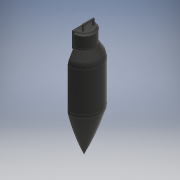
# Autodesk Inventor part: noze-cone
Saved by Autodesk Inventor 2017 (Build 210142000, 142)
## iProperties
Created: 2020-06-18
Part Number: noze-cone
Material: Polycarbonate, Clear
Document SubType Name: Modeling
Designer: HAYNIE R&D
Density: 1.2 g/cm^3
Appearance: Smooth - Black
Mass: 19.1961 g
Surface Area: 332.143 cm^2
Volume: 18.1095 cm^3
Author: HAYNIE R&D
Autodesk Inventor part; units mm, degrees
ref_plane "YZ Plane" through (0, 0, 0) normal (1, 0, 0) x (0, 1, 0)
ref_plane "XZ Plane" through (0, 0, 0) normal (0, 1, 0) x (-1, 0, 0)
ref_plane "XY Plane" through (0, 0, 0) normal (0, 0, 1) x (1, 0, 0)
sketch "Sketch1" plane through (0, 0, 0) normal (1, 0, 0) x (0, 1, 0)
  line L0 (0, 0) -> (0, -200)
  line L1 (17.75, -33.271) -> (27.75, -50.5915)
  line L2 (27.75, -50.5915) -> (27.75, -125.5915)
  line L3 (16.75, -33.271) -> (26.75, -50.5915)
  line L4 (16.75, -33.271) -> (36.75, -33.271) construction
  line L5 (26.75, -50.5915) -> (26.75, -125.5915)
  line L6 (17.75, -33.271) -> (17.75, -13.271)
  line L7 (16.75, -13.271) -> (32.074, -13.271) construction
  line L8 (17.75, -13.271) -> (33.074, -13.271) construction
  line L9 (17.75, -13.271) -> (33.074, -13.271) construction
  line L10 (16.75, -13.271) -> (31.4966, -13.271) construction
  line L11 (16.75, -33.271) -> (16.75, -14.271)
  line L12 (16.75, -14.271) -> (0, -14.271)
  line L13 (17.75, -13.271) -> (0, -13.271)
  arc A0 (0, -200) -> (27.75, -125.5915) centre (-356.6732, -24.6031) ccw
  line L14 (0, -200) -> (0, -199)
  arc A1 (0, -199) -> (26.75, -125.5915) centre (-482.9464, 18.5633) ccw
  line L15 (0, -200) -> (0, -199)
  point P0 (0, -1)
  dimension "d0" = 200
  dimension "d7" = 75
  dimension "d31" = 19
  constraints: 32 end point, 5 horizontal, 5 point on line, 5 vertical, 4 point on circle, 2 centre point, 1 collinear, 1 equal length, 1 perpendicular
  measures "d0" distance of L0.start L0.end
  measures "d7" distance of L1.end L2.end
  measures "d31" distance of L3.start L11.end
revolve "Revolution2" add sketch "Sketch1" angle 360 about axis through (0, 0, 0) along (0, 0, -1) contours L13 L6 L1 L2 A0 L0 A1 L5 L3 L11 L12
fillet "Fillet5" radius 5 1 edges at (0, -17.75, -33.271)
sketch "Sketch4" plane through (0, 0, -13.271) normal (0, 0, 1) x (1, 0, 0)
  circle A0 centre (0, 0) radius 15
  dimension "d36" = 30
  constraints: 1 centre point, 1 coincident
  measures "d36" diameter of A0
extrude "Extrusion2" add sketch "Sketch4" along normal blind 3.27
split "Split3" plane through (0, 0, 0) removes the side toward (-1, 0, 0)
fillet "Fillet8" radius 20 1 edges at (27.75, 0, -50.5915)
fillet "Fillet9" radius 25 1 edges at (27.75, 0, -125.5915)
fillet "Fillet10" radius 10 1 edges at (15, 0, -13.271)
sketch "Sketch8" plane through (0, 0, -10.001) normal (0, 0, 1) x (1, 0, 0)
  line L0 (8, -10) -> (6, -10)
  line L1 (6, -10) -> (6, -8)
  line L2 (6, -8) -> (8, -8)
  line L3 (8, -8) -> (8, -10)
  line L4 (8, 8) -> (6, 8)
  line L5 (6, 8) -> (6, 10)
  line L6 (6, 10) -> (8, 10)
  line L7 (8, 10) -> (8, 8)
  point P0 (0, 0)
  dimension "d49" = 16
  constraints: 16 end point, 4 parallel, 2 horizontal, 2 perpendicular
  measures "d49" distance of L4.end L1.end
extrude "Extrusion5" add sketch "Sketch8" along normal blind 10
sketch "Sketch9" plane through (0, 0, -0.001) normal (0, 0, 1) x (1, 0, 0)
  line L0 (6, 10) -> (8, 10) projected
  line L1 (8, -10) -> (6, -10)
  line L2 (6, -10) -> (6, 10)
  line L3 (6, 10) -> (8, 10)
  line L4 (8, 10) -> (8, -10)
  point P0 (0, 0)
  constraints: 8 end point, 2 parallel, 1 horizontal, 1 perpendicular
extrude "Extrusion6" add sketch "Sketch9" against normal blind 2
sketch "Sketch10" plane through (0, -27.75, -122.3091) normal (-1, 0, 0) x (0, 0, 1)
  line L0 (36.2789, 15.25) -> (-16.7211, 15.25)
  line L1 (-16.7211, 15.25) -> (-16.7211, 40.25)
  line L2 (-16.7211, 40.25) -> (36.2789, 40.25)
  line L3 (36.2789, 40.25) -> (36.2789, 15.25)
  line L4 (-3.2823, 1) -> (71.7177, 1) projected
  line L5 (71.7177, 54.5) -> (-3.2823, 54.5) projected
  point P0 (122.3091, 27.75)
  point P1 (-6.3725, 1)
  point P2 (-6.3725, 54.5)
  dimension "d56" = 53
  dimension "d57" = 25
  dimension "d80" = 14.25
  dimension "d81" = 14.25
  constraints: 8 end point, 2 parallel, 1 horizontal, 1 perpendicular
  measures "d56" distance of L1.end L2.end
  measures "d57" distance of L0.end L1.end
  measures "d80" distance between parallel lines of L0 L4
  measures "d81" distance between parallel lines of L5 L2
extrude "Extrusion7" add sketch "Sketch10" against normal blind 5 separate body
sketch "Sketch11" plane through (0, -27.75, -122.3091) normal (-1, 0, 0) x (0, 0, 1)
  line L0 (108.0382, 15) -> (81.5382, 15)
  line L1 (81.5382, 15) -> (81.5382, 41.5)
  line L2 (81.5382, 41.5) -> (108.0382, 41.5)
  line L3 (108.0382, 41.5) -> (108.0382, 15)
  line L4 (108.0382, 11) -> (108.0382, 44.5) projected
  line L5 (89.0382, 11) -> (108.0382, 11) projected
  line L6 (108.0382, 44.5) -> (89.0382, 44.5) projected
  point P0 (122.3091, 27.75)
  dimension "d65" = 26.5
  dimension "d66" = 26.5
  dimension "d77" = 0
  dimension "d78" = 4
  dimension "d79" = 3
  constraints: 8 end point, 2 parallel, 1 horizontal, 1 perpendicular
  measures "d65" distance of L1.end L2.end
  measures "d66" distance of L0.end L1.end
  measures "d77" distance between parallel lines of L4 L3
  measures "d78" distance between parallel lines of L0 L5
  measures "d79" distance between parallel lines of L6 L2
extrude "Extrusion8" add sketch "Sketch11" against normal blind 7.5 and the other way blind 7.5 separate body
shell "Shell4" thickness 1 removed faces 1 at (-7.5, 4.9167, -31.9376) bodies 3
shell "Shell5" thickness 1 removed faces 1 at (0, 4.1667, -121.3636) bodies 2
sketch "Sketch12" plane through (6.5, -11.75, -15.271) normal (-1, 0, 0) x (0, 0, 1)
  line L0 (-28, 12) -> (-31, 12)
  line L1 (-31, 12) -> (-31, 16)
  line L2 (-31, 16) -> (-28, 16)
  line L3 (-28, 16) -> (-28, 12)
  point P0 (15.271, 11.75)
  constraints: 8 end point, 2 parallel, 1 horizontal, 1 perpendicular
extrude "Extrusion9" cut sketch "Sketch12" along normal blind 15 bodies 3
move or copy body "Move Body1" bodies to move or copy 2 copy no translate (0, 0, 27.5)
move or copy body "Move Body2" bodies to move or copy 2 copy no translate (18, 0, 0)
chamfer "Chamfer1" distance 2 angle 45 1 edges at (26.75, 0, -50.5915)
chamfer "Chamfer2" distance 2 angle 45 1 edges at (26.75, 0, -125.5915)
sketch "Sketch15" plane through (6.5, -11.75, -15.271) normal (-1, 0, 0) x (0, 0, 1)
  circle A0 centre (-22, 22) radius 2.5
  circle A1 centre (-2.5545, 22) radius 2.5
  circle A2 centre (-22, 2.5015) radius 2.5
  circle A3 centre (-2.5545, 2.5015) radius 2.5
  point P0 (15.271, 11.75)
  dimension "d99" = 5
  dimension "d102" = 5
  dimension "d103" = 5
  dimension "d104" = 5
  constraints: 4 centre point
  measures "d99" diameter of A0
  measures "d102" diameter of A1
  measures "d103" diameter of A2
  measures "d104" diameter of A3
extrude "Extrusion11" add sketch "Sketch15" against normal blind 15 bodies 3
combine bodies "Combine2" operation type add bodies to combine 3 1
delete faces "Delete Face2" heal yes whole lump no faces at (18.7694, -11.7482, -17.783) (21.5, -9.4705, -17.2017)
delete faces "Delete Face3" heal yes whole lump no faces at (18.0789, -9.0231, -34.7811) (21.5, -8.1162, -37.7518)
delete faces "Delete Face4" heal yes whole lump no faces at (18.4508, 12.7496, -17.7824) (21.5, 8.6707, -17.5396)
delete faces "Delete Face5" heal yes whole lump no faces at (19.2552, 12.0927, -35.5814) (21.5, 10.8026, -36.6472)
sketch "Sketch16" plane through (22, -11.5, -59.5302) normal (-1, 0, 0) x (0, 0, 1)
  circle A0 centre (-48.5072, 20.4617) radius 2.5
  circle A1 centre (-2.5545, 20.4919) radius 2.5
  circle A2 centre (-2.5068, 2.512) radius 2.5
  circle A3 centre (-48.5316, 2.5218) radius 2.5
  circle A4 centre (-25, 11.5) radius 2.5
  point P0 (59.5302, 11.5)
  dimension "d107" = 5
  dimension "d108" = 5
  dimension "d109" = 5
  dimension "d110" = 5
  dimension "d111" = 5
  constraints: 5 centre point
  measures "d107" diameter of A0
  measures "d108" diameter of A1
  measures "d109" diameter of A2
  measures "d110" diameter of A3
  measures "d111" diameter of A4
extrude "Extrusion12" add sketch "Sketch16" against normal blind 15 bodies 2
sketch "Sketch18" plane through (0, -15, -10.001) normal (-1, 0, 0) x (0, 0, 1)
  line L0 (-33, 32) -> (-3, 32)
  line L1 (-3, 32) -> (-3, 0)
  line L2 (-3, 0) -> (-33, 0)
  line L3 (-33, 0) -> (-33, 32)
  point P0 (10.001, 15)
  constraints: 8 end point, 2 parallel, 1 horizontal, 1 perpendicular
extrude "Extrusion13" cut sketch "Sketch18" along normal blind 15 bodies 2
sketch "Sketch19" plane through (0, -15, -10.001) normal (-1, 0, 0) x (0, 0, 1)
  line L0 (-32, 16) -> (-28, 16)
  line L1 (-28, 16) -> (-28, 14)
  line L2 (-28, 14) -> (-32, 14)
  line L3 (-32, 14) -> (-32, 16)
  point P0 (10.001, 15)
  constraints: 8 end point, 2 parallel, 1 horizontal, 1 perpendicular
extrude "Extrusion14" cut sketch "Sketch19" against normal blind 6 bodies 2
sketch "Sketch20" plane through (18, -12.5, -58.5302) normal (-1, 0, 0) x (0, 0, 1)
  line L0 (-54, 14.5) -> (-54, 19)
  line L1 (-54, 19) -> (-59, 19)
  line L2 (-59, 19) -> (-59, 14.5)
  line L3 (-59, 14.5) -> (-59, 10)
  line L4 (-59, 10) -> (-54, 10)
  line L5 (-54, 10) -> (-54, 14.5)
  point P0 (58.5302, 12.5)
  dimension "d118" = 4.5
  dimension "d119" = 4.5
  constraints: 12 end point, 4 perpendicular, 1 point on line, 1 vertical
  measures "d118" distance of L0.start L0.end
  measures "d119" distance of L2.end L3.end
extrude "Extrusion15" cut sketch "Sketch20" against normal blind 4 and the other way blind 5 bodies 2
combine bodies "Combine4" operation type add bodies to combine 2 3
delete faces "Delete Face8" heal yes whole lump no faces at (33.0883, -11.4782, -108.0625) (23.9845, -6.4782, -108.0759) (37, -9.592, -107.8805) (33.0909, 11.4616, -108.0222) (23.9859, 6.4618, -108.0627) (37, 7.7952, -107.6465) (33.8792, 2.4993, -84.5876) (24.25, 0.2244, -87.0202) (37, -1.178, -84.2347) (33.0868, -11.488, -62.0373) (23.9837, -6.488, -62.0512) (37, -9.3753, -62.7749) (33.0863, 11.4918, -62.0699) (23.9833, 6.492, -62.1087) (37, 8.4393, -62.1175)
sketch "Sketch21" plane through (0, -15, -10.001) normal (-1, 0, 0) x (0, 0, 1)
  line L0 (-134, 23.5) -> (-112, 23.5)
  line L1 (-112, 23.5) -> (-112, 6.5)
  line L2 (-112, 6.5) -> (-134, 6.5)
  line L3 (-134, 6.5) -> (-134, 23.5)
  line L4 (-42.5905, 41.75) -> (-113.5905, 41.75) projected
  line L5 (-113.5905, -11.75) -> (-42.5905, -11.75) projected
  point P0 (10.001, 15)
  dimension "d124" = 22
  dimension "d125" = 17
  dimension "d126" = 18.25
  dimension "d127" = 18.25
  constraints: 8 end point, 2 parallel, 1 horizontal, 1 perpendicular
  measures "d124" distance of L1.end L2.end
  measures "d125" distance of L0.end L1.end
  measures "d126" distance between parallel lines of L4 L0
  measures "d127" distance between parallel lines of L5 L2
extrude "Extrusion16" add sketch "Sketch21" against normal blind 3 separate body
shell "Shell6" thickness 1 removed faces 1 at (0, 2.8333, -136.6676) bodies 4
sketch "Sketch22" plane through (2, -7.5, -143.001) normal (-1, 0, 0) x (0, 0, 1)
  circle A0 centre (10, 7.5) radius 3.75
  point P0 (143.001, 7.5)
  dimension "d131" = 7.5
  constraints: 1 centre point
  measures "d131" diameter of A0
extrude "Extrusion17" add sketch "Sketch22" against normal blind 25 bodies 4
combine bodies "Combine5" operation type add bodies to combine 4 2
delete faces "Delete Face9" heal yes whole lump no faces at (27, 0.8166, -132.8503) (26.2165, -0.484, -136.7196)
body "Solid6"
